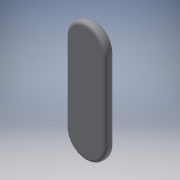
# Autodesk Inventor part: cap
Saved by Autodesk Inventor 2016 (Build 200138000, 138)
## iProperties
Created: 2016-02-14
Part Number: cap
Material: Generic
Document SubType Name: Modeling
Designer: Margret
Density: 1 g/cm^3
Appearance: Default
Author: Margret
Autodesk Inventor part; units mm, degrees
ref_plane "YZ Plane" through (0, 0, 0) normal (1, 0, 0) x (0, 1, 0)
ref_plane "XZ Plane" through (0, 0, 0) normal (0, 1, 0) x (-1, 0, 0)
ref_plane "XY Plane" through (0, 0, 0) normal (0, 0, 1) x (1, 0, 0)
ref_plane "Work Plane1" through (0, 0, 0) normal (0, 0, 1) x (1, 0, 0)
sketch "Sketch1" plane through (0, 0, 0) normal (0, 0, 1) x (1, 0, 0)
  arc A0 (20.3917, -80.7036) -> (21.6617, -79.4336) centre (20.3917, -79.4336) ccw projected
  line L0 (21.6617, -79.4336) -> (21.6617, -76.6142) projected
  arc A1 (21.6617, -76.6142) -> (20.3917, -75.3442) centre (20.3917, -76.6142) ccw projected
  line L1 (20.3917, -75.3442) -> (-1.8333, -75.3442) projected
  arc A2 (-1.8333, -75.3442) -> (-3.1033, -76.6142) centre (-1.8333, -76.6142) ccw projected
  line L2 (-3.1033, -76.6142) -> (-3.1033, -81.3894) projected
  arc A3 (-4.3733, -82.6594) -> (-3.1033, -81.3894) centre (-4.3733, -81.3894) ccw projected
  line L3 (-4.3733, -82.6594) -> (-7.8023, -82.6594) projected
  arc A4 (-7.8023, -82.6594) -> (-9.0723, -83.9294) centre (-7.8023, -83.9294) ccw projected
  line L4 (-9.0723, -83.9294) -> (-9.0723, -88.3998) projected
  arc A5 (-9.0723, -88.3998) -> (-7.8023, -89.6698) centre (-7.8023, -88.3998) ccw projected
  line L5 (-7.8023, -89.6698) -> (-3.3319, -89.6698) projected
  arc A6 (-3.3319, -89.6698) -> (-2.0619, -88.3998) centre (-3.3319, -88.3998) ccw projected
  line L6 (-2.0619, -88.3998) -> (-2.0619, -85.5109) projected
  arc A7 (-0.9806, -84.255) -> (-2.0619, -85.5109) centre (-0.7919, -85.5109) ccw projected
  arc A8 (-0.9806, -84.255) -> (4.2373, -80.7036) centre (-2.0619, -77.0575) ccw projected
  line L7 (4.2373, -80.7036) -> (20.3917, -80.7036) projected
  arc A9 (21.6617, -2.5224) -> (20.3917, -1.2524) centre (20.3917, -2.5224) ccw projected
  line L8 (4.2373, -1.2524) -> (20.3917, -1.2524) projected
  arc A10 (4.2373, -1.2524) -> (-0.9806, 2.299) centre (-2.0619, -4.8985) ccw projected
  arc A11 (-2.0619, 3.5549) -> (-0.9806, 2.299) centre (-0.7919, 3.5549) ccw projected
  line L9 (-2.0619, 6.4438) -> (-2.0619, 3.5549) projected
  arc A12 (-2.0619, 6.4438) -> (-3.3319, 7.7138) centre (-3.3319, 6.4438) ccw projected
  line L10 (-7.8023, 7.7138) -> (-3.3319, 7.7138) projected
  arc A13 (-7.8023, 7.7138) -> (-9.0723, 6.4438) centre (-7.8023, 6.4438) ccw projected
  line L11 (-9.0723, 1.9734) -> (-9.0723, 6.4438) projected
  arc A14 (-9.0723, 1.9734) -> (-7.8023, 0.7034) centre (-7.8023, 1.9734) ccw projected
  line L12 (-4.3733, 0.7034) -> (-7.8023, 0.7034) projected
  arc A15 (-3.1033, -0.5666) -> (-4.3733, 0.7034) centre (-4.3733, -0.5666) ccw projected
  line L13 (-3.1033, -5.3418) -> (-3.1033, -0.5666) projected
  arc A16 (-3.1033, -5.3418) -> (-1.8333, -6.6118) centre (-1.8333, -5.3418) ccw projected
  line L14 (20.3917, -6.6118) -> (-1.8333, -6.6118) projected
  arc A17 (20.3917, -6.6118) -> (21.6617, -5.3418) centre (20.3917, -5.3418) ccw projected
  line L15 (21.6617, -2.5224) -> (21.6617, -5.3418) projected
  arc A18 (20.3917, -81.9736) -> (22.9317, -79.4336) centre (20.3917, -79.4336) ccw
  line L16 (22.9317, -79.4336) -> (22.9317, -76.6142)
  arc A19 (22.9317, -76.6142) -> (20.3917, -74.0742) centre (20.3917, -76.6142) ccw
  line L17 (20.3917, -74.0742) -> (-1.8333, -74.0742)
  arc A20 (-1.8333, -74.0742) -> (-4.3733, -76.6142) centre (-1.8333, -76.6142) ccw
  line L18 (-4.3733, -76.6142) -> (-4.3733, -81.3894)
  line L19 (-4.3733, -81.3894) -> (-7.8023, -81.3894)
  arc A21 (-7.8023, -81.3894) -> (-10.3423, -83.9294) centre (-7.8023, -83.9294) ccw
  line L20 (-10.3423, -83.9294) -> (-10.3423, -88.3998)
  arc A22 (-10.3423, -88.3998) -> (-7.8023, -90.9398) centre (-7.8023, -88.3998) ccw
  line L21 (-7.8023, -90.9398) -> (-3.3319, -90.9398)
  arc A23 (-3.3319, -90.9398) -> (-0.7919, -88.3998) centre (-3.3319, -88.3998) ccw
  line L22 (-0.7919, -88.3998) -> (-0.7919, -85.5109)
  arc A24 (-0.7919, -85.5109) -> (4.9314, -81.9736) centre (-2.0619, -77.0575) ccw
  line L23 (4.9314, -81.9736) -> (20.3917, -81.9736)
  arc A25 (-4.3733, -5.3418) -> (-1.8333, -7.8818) centre (-1.8333, -5.3418) ccw
  line L24 (-4.3733, -5.3418) -> (-4.3733, -0.5666)
  line L25 (-4.3733, -0.5666) -> (-7.8023, -0.5666)
  arc A26 (-10.3423, 1.9734) -> (-7.8023, -0.5666) centre (-7.8023, 1.9734) ccw
  line L26 (-10.3423, 1.9734) -> (-10.3423, 6.4438)
  arc A27 (-7.8023, 8.9838) -> (-10.3423, 6.4438) centre (-7.8023, 6.4438) ccw
  line L27 (-7.8023, 8.9838) -> (-3.3319, 8.9838)
  arc A28 (-0.7919, 6.4438) -> (-3.3319, 8.9838) centre (-3.3319, 6.4438) ccw
  line L28 (-0.7919, 6.4438) -> (-0.7919, 3.5549)
  arc A29 (4.9314, 0.0176) -> (-0.7919, 3.5549) centre (-2.0619, -4.8985) ccw
  line L29 (4.9314, 0.0176) -> (20.3917, 0.0176)
  arc A30 (22.9317, -2.5224) -> (20.3917, 0.0176) centre (20.3917, -2.5224) ccw
  line L30 (22.9317, -2.5224) -> (22.9317, -5.3418)
  arc A31 (20.3917, -7.8818) -> (22.9317, -5.3418) centre (20.3917, -5.3418) ccw
  line L31 (20.3917, -7.8818) -> (-1.8333, -7.8818)
  line L32 (6.2947, -102.4206) -> (6.2947, 20.4646) construction
  line L33 (26.7417, -81.9736) -> (26.7417, 0.0176)
  line L34 (-14.1523, 0.0176) -> (-14.1523, -81.9736)
  arc A32 (-14.1523, -81.9736) -> (26.7417, -81.9736) centre (6.2947, -81.9736) ccw
  arc A33 (26.7417, 0.0176) -> (-14.1523, 0.0176) centre (6.2947, 0.0176) ccw
  point P0 (0, 0)
  point P1 (6.2947, -40.978)
  dimension "d0" = 1.27
  dimension "d1" = 1.27
  dimension "d2" = 3.81
  dimension "d3" = 3.81
  dimension "d4" = 33.0962
  dimension "d5" = 33.0962
  constraints: 40 end point, 34 point on circle, 16 centre point, 4 tangent, 3 point on line, 1 midpoint, 1 parallel, 1 vertical, 28 other
  measures "d0" distance between parallel lines of L17 L1
  measures "d1" distance between parallel lines of L31 L14
  measures "d2" distance between parallel lines of L34 L20
  measures "d3" distance between parallel lines of L33 L16
  measures "d4" distance from line of L17 point (6.295, -40.978)
  measures "d5" distance from line of point (6.295, -40.978) L31
extrude "Extrusion1" add sketch "Sketch1" against normal blind 6.35 contours A32 L34 A33 L33
sketch "Sketch2" plane through (0, 0, 0) normal (0, 0, 1) x (1, 0, 0)
  line L0 (20.3917, -7.8818) -> (-1.8333, -7.8818) projected
  arc A0 (-4.3733, -5.3418) -> (-1.8333, -7.8818) centre (-1.8333, -5.3418) ccw projected
  line L1 (-4.3733, -5.3418) -> (-4.3733, -0.5666) projected
  line L2 (-4.3733, -0.5666) -> (-7.8023, -0.5666) projected
  arc A1 (-10.3423, 1.9734) -> (-7.8023, -0.5666) centre (-7.8023, 1.9734) ccw projected
  line L3 (-10.3423, 1.9734) -> (-10.3423, 6.4438) projected
  arc A2 (-7.8023, 8.9838) -> (-10.3423, 6.4438) centre (-7.8023, 6.4438) ccw projected
  line L4 (-7.8023, 8.9838) -> (-3.3319, 8.9838) projected
  arc A3 (-0.7919, 6.4438) -> (-3.3319, 8.9838) centre (-3.3319, 6.4438) ccw projected
  line L5 (-0.7919, 6.4438) -> (-0.7919, 3.5549) projected
  arc A4 (4.9314, 0.0176) -> (-0.7919, 3.5549) centre (-2.0619, -4.8985) ccw projected
  line L6 (4.9314, 0.0176) -> (20.3917, 0.0176) projected
  arc A5 (22.9317, -2.5224) -> (20.3917, 0.0176) centre (20.3917, -2.5224) ccw projected
  line L7 (22.9317, -2.5224) -> (22.9317, -5.3418) projected
  arc A6 (20.3917, -7.8818) -> (22.9317, -5.3418) centre (20.3917, -5.3418) ccw projected
  line L8 (22.9317, -76.6142) -> (22.9317, -79.4336) projected
  arc A7 (20.3917, -81.9736) -> (22.9317, -79.4336) centre (20.3917, -79.4336) ccw projected
  line L9 (20.3917, -81.9736) -> (4.9314, -81.9736) projected
  arc A8 (-0.7919, -85.5109) -> (4.9314, -81.9736) centre (-2.0619, -77.0575) ccw projected
  line L10 (-0.7919, -85.5109) -> (-0.7919, -88.3998) projected
  arc A9 (-3.3319, -90.9398) -> (-0.7919, -88.3998) centre (-3.3319, -88.3998) ccw projected
  line L11 (-3.3319, -90.9398) -> (-7.8023, -90.9398) projected
  arc A10 (-10.3423, -88.3998) -> (-7.8023, -90.9398) centre (-7.8023, -88.3998) ccw projected
  line L12 (-10.3423, -88.3998) -> (-10.3423, -83.9294) projected
  arc A11 (-7.8023, -81.3894) -> (-10.3423, -83.9294) centre (-7.8023, -83.9294) ccw projected
  line L13 (-7.8023, -81.3894) -> (-4.3733, -81.3894) projected
  line L14 (-4.3733, -81.3894) -> (-4.3733, -76.6142) projected
  arc A12 (-1.8333, -74.0742) -> (-4.3733, -76.6142) centre (-1.8333, -76.6142) ccw projected
  line L15 (-1.8333, -74.0742) -> (20.3917, -74.0742) projected
  arc A13 (22.9317, -76.6142) -> (20.3917, -74.0742) centre (20.3917, -76.6142) ccw projected
  line L16 (26.7417, -81.9736) -> (26.7417, 0.0176) projected
  arc A14 (26.7417, 0.0176) -> (-14.1523, 0.0176) centre (6.2947, 0.0176) ccw projected
  line L17 (-14.1523, 0.0176) -> (-14.1523, -81.9736) projected
  arc A15 (-14.1523, -81.9736) -> (26.7417, -81.9736) centre (6.2947, -81.9736) ccw projected
  point P0 (0, 0)
extrude "Extrusion2" add sketch "Sketch2" along normal blind 2.54 contours L0 A0 L1 L2 A1 L3 A2 L4 A3 L5 A4 L6 A5 L7 A6 | L8 A7 L9 A8 L10 A9 L11 A10 L12 A11 L13 L14 A12 L15 A13 | A15 L17 A14 L16
fillet "Fillet1" radius 3.175 8 edges at (-14.1523, -40.978, 2.54) (6.2947, -102.4206, 2.54) (26.7417, -40.978, 2.54) (6.2947, 20.4646, 2.54) (-14.1523, -40.978, -6.35) (6.2947, 20.4646, -6.35) (26.7417, -40.978, -6.35) (6.2947, -102.4206, -6.35)
equation "\"d1\" = d0"
equation "\"d3\" = d2"
equation "\"d4\" = d5"
body "Solid1"
